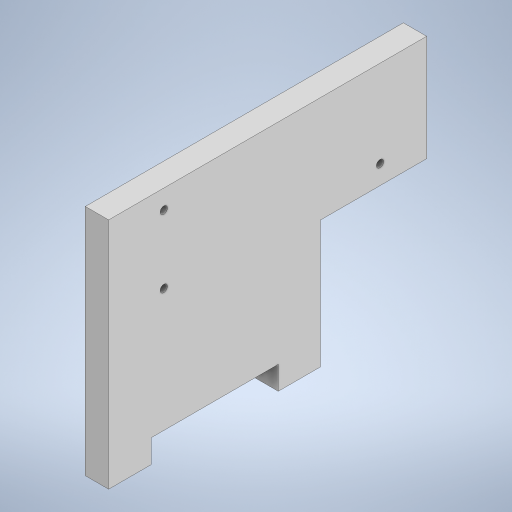
# Autodesk Inventor part: 壁
Saved by Autodesk Inventor 2024.1 (Build 281209000, 209)
## iProperties
Created: 2024-04-01
Part Number: 壁
Material: 一般
Document SubType Name: Modeling
Designer: hibik
Density: 1 g/cm^3
Appearance: 既定
Author: hibik
Autodesk Inventor part; units mm, degrees
ref_plane "YZ Plane" through (0, 0, 0) normal (1, 0, 0) x (0, 1, 0)
ref_plane "XZ Plane" through (0, 0, 0) normal (0, 1, 0) x (-1, 0, 0)
ref_plane "XY Plane" through (0, 0, 0) normal (0, 0, 1) x (1, 0, 0)
sketch "スケッチ1" plane through (0, 0, 0) normal (1, 0, 0) x (0, 1, 0)
  line L0 (0, 0) -> (30, 0)
  line L1 (30, 0) -> (30, -50) construction
  line L2 (30, -50) -> (0, -50)
  line L3 (0, -50) -> (0, 0)
  line L4 (30, 0) -> (55, 0)
  line L5 (55, 0) -> (55, -50)
  line L6 (55, -50) -> (30, -50)
  line L7 (30, -50) -> (30, 0) construction
  circle A0 centre (50.5, -13) radius 0.85
  circle A1 centre (34.5, -13) radius 0.85
  line L8 (50.5, -13) -> (34.5, -13) construction
  line L9 (0, 0) -> (5.5, 0)
  line L10 (5.5, 0) -> (5.5, -10)
  line L11 (5.5, -10) -> (0, -10)
  line L12 (0, -10) -> (0, 0)
  line L13 (0, -50) -> (5.5, -50)
  line L14 (5.5, -50) -> (5.5, -40)
  line L15 (5.5, -40) -> (0, -40)
  line L16 (0, -40) -> (0, -50)
  line L17 (34.5, -13) -> (34.5, -64) construction
  line L18 (34.5, -13) -> (85.5, -13) construction
  circle A2 centre (34.5, -64) radius 0.85
  line L19 (55, -50) -> (30, -50)
  line L20 (30, -50) -> (30, -75)
  line L21 (30, -75) -> (55, -75)
  line L22 (55, -75) -> (55, -50)
  line L23 (5.5, -10) -> (5.5, -40)
  point P0 (55, -25)
  point P1 (42.5, -13)
  point P2 (42.5, -50)
  point P3 (0, -40)
  dimension "d0" = 30
  dimension "d1" = 50
  dimension "d2" = 25
  dimension "d3" = 1.7
  dimension "d4" = 1.7
  dimension "d5" = 12
  dimension "d6" = 16
  dimension "d7" = 10
  dimension "d8" = 5.5
  dimension "d9" = 51
  dimension "d10" = 90
  dimension "d11" = 1.7
  constraints: 48 end point, 10 parallel, 7 horizontal, 6 perpendicular, 3 centre point, 3 collinear, 3 equal length, 3 midpoint, 2 coincident, 1 horizontal alignment, 1 vertical, 1 vertical alignment
  measures "d0" distance of L1.end L2.end
  measures "d1" distance of L2.end L0.start
  measures "d2" distance of L5.end L6.end
  measures "d3" diameter of A0
  measures "d4" diameter of A1
  measures "d5" vertical distance of point (55, -25) L8.start
  measures "d6" distance of L8.end L8.start
  measures "d7" distance of L9.end L10.end
  measures "d8" distance between parallel lines of L3 L10
  measures "d9" distance of L8.end L17.end
  measures "d10" angle of L17 L18
  measures "d11" diameter of A2
extrude "押し出し1" add sketch "スケッチ1" along normal blind 5.5 contours L0 L10 L11 L3 | L0 L4 L5 L6 L2 L14 L23 L10 | L15 L14 L2 L3 | L22 L21 L20 L6
